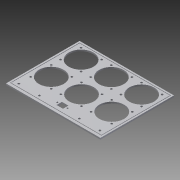
# Autodesk Inventor part: plate
Saved by Autodesk Inventor 2014 SP1 (Build 180222100, 222)
## iProperties
Created: 2016-09-05
Part Number: plate
Material: ABS Plastic
Document SubType Name: Modeling
Designer: tguillod
Density: 1.06 g/cm^3
Appearance: Smooth - White
Author: tguillod
Autodesk Inventor part; units mm, degrees
ref_plane "YZ Plane" through (0, 0, 0) normal (1, 0, 0) x (0, 1, 0)
ref_plane "XZ Plane" through (0, 0, 0) normal (0, 1, 0) x (-1, 0, 0)
ref_plane "XY Plane" through (0, 0, 0) normal (0, 0, 1) x (1, 0, 0)
sketch "Sketch1" plane through (0, 0, 0) normal (0, 0, 1) x (1, 0, 0)
  line L0 (0, 0) -> (183.5, 0)
  line L1 (183.5, 0) -> (183.5, 143)
  line L2 (183.5, 143) -> (0, 143)
  line L3 (0, 143) -> (0, 0)
  dimension "d0" = 183.5
  dimension "d1" = 143
  constraints: 8 end point, 2 parallel, 1 horizontal, 1 perpendicular
  measures "d0" distance of L1.end L2.end
  measures "d1" distance of L0.end L1.end
extrude "Extrusion1" add sketch "Sketch1" along normal blind 3
sketch "Sketch3" plane through (0, 0, 3) normal (0, 0, 1) x (1, 0, 0)
  line L0 (0, 0) -> (183.5, 0) projected
  line L1 (183.5, 0) -> (183.5, 143) projected
  line L2 (183.5, 143) -> (0, 143) projected
  line L3 (0, 143) -> (0, 0) projected
  line L4 (0, 133) -> (183.5, 133) construction
  line L5 (13, 143) -> (13, 0) construction
  line L6 (0, 93) -> (183.5, 93) construction
  line L7 (183.5, 75) -> (0, 75) construction
  line L8 (0, 35) -> (183.5, 35) construction
  line L9 (53, 143) -> (53, 0) construction
  line L10 (130.5, 143) -> (130.5, 0) construction
  line L11 (111.75, 143) -> (111.75, 0) construction
  line L12 (71.75, 143) -> (71.75, 0) construction
  line L13 (170.5, 143) -> (170.5, 0) construction
  line L14 (0, 12) -> (183.5, 12) construction
  point P0 (13, 133)
  point P1 (53, 133)
  point P2 (71.75, 133)
  point P3 (111.75, 133)
  point P4 (130.5, 133)
  point P5 (170.5, 133)
  point P6 (170.5, 93)
  point P7 (130.5, 93)
  point P8 (111.75, 93)
  point P9 (71.75, 93)
  point P10 (53, 93)
  point P11 (13, 93)
  point P12 (53, 35)
  point P13 (53, 75)
  point P14 (13, 75)
  point P15 (13, 35)
  point P16 (130.5, 35)
  point P17 (170.5, 35)
  point P18 (170.5, 75)
  point P19 (130.5, 75)
  point P20 (71.75, 75)
  point P21 (111.75, 75)
  point P22 (111.75, 35)
  point P23 (71.75, 35)
  point P24 (13, 12)
  point P25 (53, 12)
  point P26 (130.5, 12)
  point P27 (170.5, 12)
  dimension "d5" = 40
  dimension "d6" = 40
  dimension "d7" = 40
  dimension "d8" = 40
  dimension "d9" = 40
  dimension "d10" = 13
  dimension "d11" = 13
  dimension "d12" = 10
  dimension "d13" = 18
  dimension "d14" = 18.75
  dimension "d30" = 18.75
  dimension "d40" = 12
  constraints: 78 point on line, 22 end point, 9 perpendicular, 2 parallel
  measures "d5" distance between parallel lines of L9 L5
  measures "d6" distance between parallel lines of L6 L4
  measures "d7" distance between parallel lines of L8 L7
  measures "d8" distance between parallel lines of L11 L12
  measures "d9" distance between parallel lines of L13 L10
  measures "d10" distance between parallel lines of L5 L3
  measures "d11" distance between parallel lines of L1 L13
  measures "d12" distance between parallel lines of L4 L2
  measures "d13" distance between parallel lines of L7 L6
  measures "d14" distance between parallel lines of L12 L9
  measures "d30" distance between parallel lines of L10 L11
  measures "d40" distance between parallel lines of L14 L0
hole "Hole1" at (13, 133, 3) at (53, 133, 3) at (71.75, 133, 3) at (111.75, 133, 3) at (130.5, 133, 3) at (170.5, 133, 3) at (170.5, 93, 3) at (130.5, 93, 3) at (111.75, 93, 3) at (71.75, 93, 3) at (53, 93, 3) at (13, 93, 3) at (53, 35, 3) at (53, 75, 3) at (13, 75, 3) at (13, 35, 3) at (130.5, 35, 3) at (170.5, 35, 3) at (170.5, 75, 3) at (130.5, 75, 3) at (71.75, 75, 3) at (111.75, 75, 3) at (71.75, 35, 3) at (111.75, 35, 3) at (13, 12, 3) at (53, 12, 3) at (130.5, 12, 3) at (170.5, 12, 3) direction (0, 0, -1) diameter 4 end through all
sketch "Sketch4" plane through (0, 0, 3) normal (0, 0, 1) x (1, 0, 0)
  circle A0 centre (170.5, 75) radius 2 projected
  circle A1 centre (130.5, 35) radius 2 projected
  circle A2 centre (13, 75) radius 2 projected
  circle A3 centre (53, 35) radius 2 projected
  circle A4 centre (53, 93) radius 2 projected
  circle A5 centre (111.75, 93) radius 2 projected
  circle A6 centre (170.5, 93) radius 2 projected
  circle A7 centre (130.5, 133) radius 2 projected
  circle A8 centre (71.75, 133) radius 2 projected
  circle A9 centre (13, 133) radius 2 projected
  circle A10 centre (53, 133) radius 2 projected
  circle A11 centre (111.75, 133) radius 2 projected
  circle A12 centre (170.5, 133) radius 2 projected
  circle A13 centre (130.5, 93) radius 2 projected
  circle A14 centre (71.75, 93) radius 2 projected
  circle A15 centre (13, 93) radius 2 projected
  circle A16 centre (53, 75) radius 2 projected
  circle A17 centre (13, 35) radius 2 projected
  circle A18 centre (170.5, 35) radius 2 projected
  circle A19 centre (130.5, 75) radius 2 projected
  line L0 (13, 133) -> (53, 93) construction
  line L1 (71.75, 133) -> (111.75, 93) construction
  line L2 (53, 133) -> (13, 93) construction
  line L3 (71.75, 93) -> (111.75, 133) construction
  line L4 (130.5, 133) -> (170.5, 93) construction
  line L5 (170.5, 133) -> (130.5, 93) construction
  line L6 (130.5, 75) -> (170.5, 35) construction
  line L7 (170.5, 75) -> (130.5, 35) construction
  line L8 (13, 75) -> (53, 35) construction
  line L9 (53, 75) -> (13, 35) construction
  circle A20 centre (33, 113) radius 24
  circle A21 centre (91.75, 113) radius 24
  circle A22 centre (150.5, 113) radius 24
  circle A23 centre (150.5, 55) radius 24
  circle A24 centre (33, 55) radius 24
  circle A25 centre (71.75, 35) radius 2 projected
  circle A26 centre (71.75, 75) radius 2 projected
  circle A27 centre (111.75, 75) radius 2 projected
  circle A28 centre (111.75, 35) radius 2 projected
  line L10 (71.75, 75) -> (111.75, 35) construction
  line L11 (111.75, 75) -> (71.75, 35) construction
  circle A29 centre (91.75, 55) radius 24
  dimension "d22" = 48
  dimension "d23" = 48
  dimension "d24" = 48
  dimension "d25" = 48
  dimension "d26" = 48
  dimension "d29" = 48
  constraints: 24 end point, 9 perpendicular, 6 centre point, 6 midpoint, 2 parallel
  measures "d22" diameter of A20
  measures "d23" diameter of A21
  measures "d24" diameter of A22
  measures "d25" diameter of A23
  measures "d26" diameter of A24
  measures "d29" diameter of A29
extrude "Extrusion2" cut sketch "Sketch4" against normal blind 48 contours A20 | A21 | A22 | A23 | A24 | A29
sketch "Sketch5" plane through (0, 0, 3) normal (0, 0, 1) x (1, 0, 0)
  line L0 (0, 0) -> (183.5, 0) projected
  line L1 (183.5, 0) -> (183.5, 143) projected
  line L2 (183.5, 143) -> (0, 143) projected
  line L3 (0, 143) -> (0, 0) projected
  line L4 (91.75, 143) -> (91.75, 0) construction
  line L5 (85.45, 23.25) -> (98.05, 23.25)
  line L6 (98.05, 23.25) -> (98.05, 12.75)
  line L7 (98.05, 12.75) -> (85.45, 12.75)
  line L8 (85.45, 12.75) -> (85.45, 23.25)
  line L9 (85.45, 23.25) -> (98.05, 12.75) construction
  line L10 (98.05, 23.25) -> (85.45, 12.75) construction
  circle A0 centre (81.87, 18) radius 1.5
  circle A1 centre (101.63, 18) radius 1.5
  line L11 (0, 18) -> (183.5, 18) construction
  point P0 (91.75, 18)
  point P1 (91.75, 18)
  dimension "d31" = 18
  dimension "d32" = 10.5
  dimension "d33" = 12.6
  dimension "d34" = 9.88
  dimension "d35" = 9.88
  dimension "d36" = 3
  dimension "d37" = 3
  constraints: 16 end point, 6 midpoint, 5 point on line, 2 centre point, 2 parallel, 2 perpendicular, 1 horizontal
  measures "d31" distance between parallel lines of L11 L0
  measures "d32" distance of L7.end L5.start
  measures "d33" distance of L6.end L7.end
  measures "d34" distance from line of A0.centre L4
  measures "d35" distance of point (91.75, 18) A1.centre
  measures "d36" diameter of A0
  measures "d37" diameter of A1
extrude "Extrusion3" cut sketch "Sketch5" against normal blind 10 contours L5 L6 L7 L8 | A0 | A1
sketch "Sketch6" plane through (0, 0, 3) normal (0, 0, 1) x (1, 0, 0)
  line L0 (0, 0) -> (183.5, 0) projected
  line L1 (183.5, 0) -> (183.5, 143) projected
  line L2 (183.5, 143) -> (0, 143) projected
  line L3 (0, 143) -> (0, 0) projected
  line L4 (3, 140) -> (180.5, 140)
  line L5 (180.5, 140) -> (180.5, 139)
  line L6 (180.5, 139) -> (3, 139)
  line L7 (3, 139) -> (3, 140)
  line L8 (3, 139) -> (4, 139)
  line L9 (4, 139) -> (4, 5)
  line L10 (4, 5) -> (3, 5)
  line L11 (3, 5) -> (3, 139)
  line L12 (4, 5) -> (179.5, 5)
  line L13 (179.5, 5) -> (179.5, 6)
  line L14 (179.5, 6) -> (4, 6)
  line L15 (4, 6) -> (4, 5)
  line L16 (180.5, 139) -> (179.5, 139)
  line L17 (179.5, 139) -> (179.5, 6)
  line L18 (179.5, 6) -> (180.5, 6)
  line L19 (180.5, 6) -> (180.5, 139)
  line L20 (179.5, 6) -> (180.5, 6)
  line L21 (180.5, 6) -> (180.5, 5)
  line L22 (180.5, 5) -> (179.5, 5)
  line L23 (179.5, 5) -> (179.5, 6)
  dimension "d41" = 1
  dimension "d42" = 1
  dimension "d43" = 1
  dimension "d44" = 1
  dimension "d45" = 3
  dimension "d46" = 3
  dimension "d47" = 3
  dimension "d48" = 5
  constraints: 40 end point, 10 parallel, 5 horizontal, 5 perpendicular, 4 collinear
  measures "d41" distance of L4.end L5.end
  measures "d42" distance of L17.end L18.end
  measures "d43" distance of L9.end L10.end
  measures "d44" distance between parallel lines of L12 L14
  measures "d45" distance between parallel lines of L2 L4
  measures "d46" distance between parallel lines of L1 L19
  measures "d47" distance between parallel lines of L3 L11
  measures "d48" distance between parallel lines of L0 L12
extrude "Extrusion4" add sketch "Sketch6" along normal blind 1 contours L4 L5 L6 L7 | L6 L9 L10 L11 | L19 L18 L17 L6 | L21 L22 L13 L18 | L14 L13 L12 L9
equation "\"d27\" = d29"
body "Solid1"
